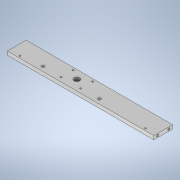
# Autodesk Inventor part: Culata
Saved by Autodesk Inventor 2020 (Build 240168000, 168)
## iProperties
Created: 2020-05-08
Part Number: Culata
Material: Aluminio 6061
Document SubType Name: Modeling
Designer: Pipi
Density: 2.7 g/cm^3
Appearance: Aluminum - Dark
Mass: 509.5 g
Surface Area: 497.713 cm^2
Volume: 188.704 cm^3
Author: Pipi
Autodesk Inventor part; units mm, degrees
ref_plane "YZ Plane" through (0, 0, 0) normal (1, 0, 0) x (0, 1, 0)
ref_plane "XZ Plane" through (0, 0, 0) normal (0, 1, 0) x (-1, 0, 0)
ref_plane "XY Plane" through (0, 0, 0) normal (0, 0, 1) x (1, 0, 0)
sketch "Boceto1" plane through (0, 0, 0) normal (0, 1, 0) x (-1, 0, 0)
  line L0 (-32, 16) -> (-32, 66)
  line L1 (-32, 66) -> (358, 66)
  line L2 (358, 66) -> (358, 16)
  line L3 (358, 16) -> (-32, 16)
  circle A0 centre (200, 39) radius 7.5
  circle A1 centre (275, 54) radius 4
  circle A2 centre (125, 54) radius 4
  line L4 (179, 60) -> (179, 18)
  line L5 (179, 18) -> (221, 18)
  line L6 (221, 18) -> (221, 60)
  line L7 (221, 60) -> (179, 60)
  circle A3 centre (184.5, 54.5) radius 2
  circle A4 centre (215.5, 54.5) radius 2
  circle A5 centre (215.5, 23.5) radius 2
  circle A6 centre (184.5, 23.5) radius 2
  circle A7 centre (174, 55) radius 2
  line L8 (169, 60) -> (179, 60)
  line L9 (200, 39) -> (195, 39)
  line L10 (195, 39) -> (200, 39)
  line L11 (200, 60) -> (200, 61)
  circle A8 centre (226, 55) radius 2
  line L12 (231, 60) -> (221, 60)
  circle A9 centre (174, 23) radius 2
  line L13 (169, 18) -> (179, 18)
  circle A10 centre (226, 23) radius 2
  line L14 (231, 18) -> (221, 18)
  circle A11 centre (330, 60.5) radius 2
  circle A12 centre (-4, 60.5) radius 2
  point P0 (0, 0)
  dimension "d0" = 50
  dimension "d1" = 390
  dimension "d2" = 15
  dimension "d4" = 8
  dimension "d5" = 8
  dimension "d6" = 15
  dimension "d7" = 75
  dimension "d8" = 75
  dimension "d91" = 4
  dimension "d92" = 4
  dimension "d93" = 4
  dimension "d94" = 4
  dimension "d95" = 31
  dimension "d96" = 31
  dimension "d97" = 31
  dimension "d98" = 31
  dimension "d99" = 5.5
  dimension "d100" = 5.5
  dimension "d101" = 5.5
  dimension "d102" = 5.5
  dimension "d103" = 5.5
  dimension "d104" = 5.5
  dimension "d106" = 4
  dimension "d112" = 5
  dimension "d113" = 5
  dimension "d115" = 42
  dimension "d116" = 12
  dimension "d117" = 12
  dimension "d142" = 4
  dimension "d143" = 4
  dimension "d144" = 5.5
  dimension "d145" = 157
  dimension "d146" = 28
  dimension "d147" = 5.5
  dimension "d148" = 28
  constraints: 30 end point, 13 centre point, 8 symmetric about line, 4 perpendicular, 3 vertical, 2 collinear, 1 horizontal, 1 midpoint, 3 other
  measures "d0" distance of L3.end L1.start
  measures "d1" distance of L1.start L1.end
  measures "d2" diameter of A0
  measures "d4" diameter of A1
  measures "d5" diameter of A2
  measures "d6" vertical distance of A1.centre L9.start
  measures "d7" horizontal distance of L9.start A1.centre
  measures "d8" horizontal distance of A2.centre L9.start
  measures "d91" diameter of A3
  measures "d92" diameter of A4
  measures "d93" diameter of A5
  measures "d94" diameter of A6
  measures "d95" distance of A6.centre A3.centre
  measures "d96" distance of A3.centre A4.centre
  measures "d97" distance of A4.centre A5.centre
  measures "d98" distance of A6.centre A5.centre
  measures "d99" distance from line of L4 A3.centre
  measures "d100" distance from line of L7 A4.centre
  measures "d101" distance from line of L4 A6.centre
  measures "d102" distance from line of L5 A5.centre
  measures "d103" distance from line of L5 A6.centre
  measures "d104" distance from line of A5.centre L6
  measures "d106" diameter of A7
  measures "d112" distance from line of A7.centre L4
  measures "d113" distance from line of L8 A7.centre
  measures "d115" distance between parallel lines of L14 L12
  measures "d116" distance from line of L1 A2.centre
  measures "d117" distance from line of L1 A1.centre
  measures "d142" diameter of A11
  measures "d143" diameter of A12
  measures "d144" distance from line of L1 A11.centre
  measures "d145" distance from line of L0 A2.centre
  measures "d146" distance from line of L2 A11.centre
  measures "d147" distance from line of L1 A12.centre
  measures "d148" distance from line of L0 A12.centre
extrude "Extrusión1" add sketch "Boceto1" along normal blind 10 contours L0 L1 L2 L3 | L7 L6 L5 L4 | A3 | A4 | A5 | A6
sketch "Boceto6" plane through (32, 0, 66) normal (1, 0, 0) x (0, 0, -1)
  line L0 (0, 0) -> (0, 10) projected
  line L1 (0, 5) -> (50, 5)
  line L2 (50, 0) -> (50, 10) projected
  line L3 (50, 5) -> (40, 5)
  line L4 (0, 5) -> (10, 5)
  circle A0 centre (10, 5) radius 3
  circle A1 centre (40, 5) radius 3
  point P0 (66, 0)
  dimension "d35" = 10
  dimension "d36" = 6
  dimension "d37" = 6
  dimension "d119" = 10
  constraints: 6 end point, 2 centre point, 2 coincident, 2 midpoint, 2 point on line
  measures "d35" distance of L1.start L4.end
  measures "d36" diameter of A0
  measures "d37" diameter of A1
  measures "d119" distance of L1.end L3.end
hole "Agujero1" at (32, 5, 56) at (32, 5, 26) direction (-1, 0, 0) diameter 6 depth 15 tip angle 118
sketch "Boceto8" plane through (-358, 0, 16) normal (-1, 0, 0) x (0, 0, 1)
  line L0 (50, 0) -> (50, 10) projected
  line L1 (50, 5) -> (37.5, 5)
  line L2 (37.5, 5) -> (12.5, 5)
  circle A0 centre (40, 5) radius 3 projected
  circle A1 centre (40, 5) radius 3
  circle A2 centre (12.5, 5) radius 3
  point P0 (-16, 0)
  dimension "d58" = 12.5
  dimension "d59" = 25
  dimension "d60" = 6
  dimension "d61" = 6
  constraints: 4 end point, 2 centre point, 2 coincident, 1 horizontal, 1 midpoint, 1 point on line
  measures "d58" distance of L1.start L1.end
  measures "d59" distance of L1.end L2.end
  measures "d60" diameter of A1
  measures "d61" diameter of A2
hole "Agujero3" at (-358, 5, 53.5) at (-358, 5, 28.5) direction (1, 0, 0) diameter 6 depth 15 tip angle 118
thread "Rosca1" size "M6x1" class "6H" standard "ISO Metric profile" length 430
thread "Rosca2" size "M6x1" class "6H" standard "ISO Metric profile" length 430
thread "Rosca3" size "M6x1" class "6H" standard "ISO Metric profile" length 430
thread "Rosca4" size "M6x1" class "6H" standard "ISO Metric profile" length 430
thread "Rosca5" size "M4x0.7" class "6H" standard "ISO Metric profile" length 22
thread "Rosca6" size "M4x0.7" class "6H" standard "ISO Metric profile" length 22
thread "Rosca7" size "M4x0.7" class "6H" standard "ISO Metric profile" length 22
thread "Rosca8" size "M4x0.7" class "6H" standard "ISO Metric profile" length 922
thread "Rosca9" size "M4x0.7" class "6H" standard "ISO Metric profile" length 100
thread "Rosca10" size "M4x0.7" class "6H" standard "ISO Metric profile" length 100
equation "\"d35\" = d119"
